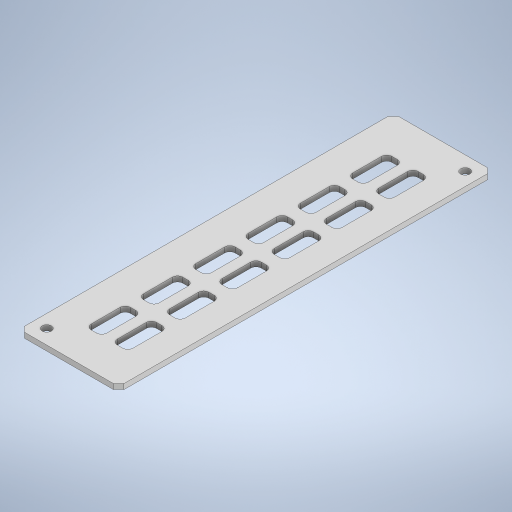
# Autodesk Inventor part: battery case Lid
Saved by Autodesk Inventor 2024 (Build 280153020, 153B)
## iProperties
Created: 2024-02-15
Part Number: battery case Lid
Material: Generic
Document SubType Name: Modeling
Designer: scottst
Density: 1 g/cm^3
Appearance: Default
Author: scottst
Autodesk Inventor part; units mm, degrees
ref_plane "YZ Plane" through (0, 0, 0) normal (1, 0, 0) x (0, 1, 0)
ref_plane "XZ Plane" through (0, 0, 0) normal (0, 1, 0) x (-1, 0, 0)
ref_plane "XY Plane" through (0, 0, 0) normal (0, 0, 1) x (1, 0, 0)
sketch "Sketch1" plane through (0, 0, 0) normal (0, 1, 0) x (-1, 0, 0)
  line L0 (-19, 71.5) -> (19, 71.5)
  line L1 (19, 71.5) -> (19, -71.5)
  line L2 (19, -71.5) -> (-19, -71.5)
  line L3 (-19, -71.5) -> (-19, 71.5)
  line L4 (-19, 71.5) -> (19, -71.5) construction
  line L5 (19, 71.5) -> (-19, -71.5) construction
  point P0 (0, 0)
  dimension "d0" = 38
  dimension "d1" = 143
  constraints: 12 end point, 2 midpoint, 2 parallel, 1 horizontal, 1 perpendicular
  measures "d0" distance of L1.end L2.end
  measures "d1" distance of L0.end L1.end
extrude "Extrusion1" add sketch "Sketch1" along normal blind 2
sketch "Sketch2" plane through (0, 2, 0) normal (0, 1, 0) x (1, 0, 0)
  line L0 (-19, -71.5) -> (-19, -66) construction
  line L1 (-19, -66) -> (-14, -66) construction
  line L2 (-19, -66) -> (-14, -66) construction
  line L3 (19, 71.5) -> (-19, 71.5) construction
  line L4 (19, 71.5) -> (19, 66) construction
  line L5 (19, 66) -> (14, 66) construction
  line L6 (19, 66) -> (24, 66) construction
  circle A0 centre (14, 66) radius 1.75
  circle A1 centre (-14, -66) radius 1.75
  point P0 (0, 0)
  dimension "d4" = 5.5
  dimension "d7" = 5
  dimension "d8" = 0
  dimension "d9" = 5.5
  dimension "d12" = 180
  dimension "d13" = 3.5
  dimension "d14" = 3.5
  constraints: 12 end point, 3 horizontal, 2 centre point, 2 coincident, 2 collinear
  measures "d4" distance of L0.start L0.end
  measures "d7" distance of L0.end L1.end
  measures "d8" distance between parallel lines of L1 L2
  measures "d9" distance of L3.start L4.end
  measures "d12" angle of L5 L6
  measures "d13" diameter of A0
  measures "d14" diameter of A1
extrude "Extrusion2" cut sketch "Sketch2" against normal blind 14.75
sketch "Sketch3" plane through (0, 0, 0) normal (0, -1, 0) x (1, 0, 0)
  line L0 (-14.75, 51.7235) -> (14.75, 51.7235)
  line L1 (14.75, 51.7235) -> (14.75, -51.7235)
  line L2 (14.75, -51.7235) -> (-14.75, -51.7235)
  line L3 (-14.75, -51.7235) -> (-14.75, 51.7235)
  line L4 (-14.75, 51.7235) -> (14.75, -51.7235) construction
  line L5 (14.75, 51.7235) -> (-14.75, -51.7235) construction
  line L6 (12.75, -49.7235) -> (12.75, 49.7235)
  line L7 (12.75, 49.7235) -> (-12.75, 49.7235)
  line L8 (-12.75, 49.7235) -> (-12.75, -49.7235)
  line L9 (-12.75, -49.7235) -> (12.75, -49.7235)
  line L10 (-14.75, 49.7235) -> (14.75, 49.7235)
  line L11 (-14.75, -49.7235) -> (14.75, -49.7235)
  line L12 (-14.75, 0) -> (-14.75, -25)
  line L13 (-14.75, -25) -> (14.75, -25)
  line L14 (-14.75, 0) -> (-14.75, 25)
  line L15 (-14.75, 25) -> (14.75, 25)
  point P0 (0, 0)
  point P1 (-12.75, -25)
  point P2 (12.75, -25)
  point P3 (12.75, 25)
  point P4 (-12.75, 25)
  dimension "d17" = 29.5
  dimension "d18" = 2
  dimension "d19" = 25
  dimension "d20" = 25
  constraints: 32 end point, 10 point on line, 4 parallel, 4 perpendicular, 3 midpoint, 1 horizontal, 3 other
  measures "d17" distance of L1.end L2.end
  measures "d18" distance between parallel lines of L1 L6
  measures "d19" distance of L12.start L12.end
  measures "d20" distance of L12.start L14.end
extrude "Extrusion3" add sketch "Sketch3" along normal blind 2 contours L10 L8 L15 L3 | L1 L15 L6 L10 | L1 L11 L6 L13 | L13 L8 L11 L3
sketch "Sketch4" plane through (0, 0, 0) normal (0, -1, 0) x (1, 0, 0)
  line L0 (-19, 71.5) -> (19, 71.5) construction
  line L1 (0, 71.5) -> (0, -71.5) construction
  line L2 (19, -71.5) -> (-19, -71.5) construction
  line L3 (3, 16) -> (3, 5) construction
  line L4 (-3, 71.5) -> (-3, -71.5) construction
  line L5 (-9, 71.5) -> (-9, -71.5) construction
  line L6 (9, 16) -> (9, -71.5) construction
  line L7 (19, 71.5) -> (19, -71.5) construction
  line L8 (19, 0) -> (-19, 0) construction
  line L9 (19, 3) -> (5, 3) construction
  line L10 (3, 3) -> (7, 3)
  line L11 (9, 5) -> (9, 18)
  line L12 (7, 18) -> (5, 18)
  line L13 (3, 18) -> (3, 3)
  arc A0 (5, 18) -> (3, 16) centre (5, 16) ccw
  arc A1 (9, 16) -> (7, 18) centre (7, 16) ccw
  arc A2 (7, 3) -> (9, 5) centre (7, 5) ccw
  arc A3 (3, 5) -> (5, 3) centre (5, 5) ccw
  point P0 (0, 0)
  point P1 (9, 3)
  dimension "d23" = 3
  dimension "d24" = 3
  dimension "d25" = 6
  dimension "d26" = 6
  dimension "d27" = 3
  dimension "d28" = 15
  dimension "d29" = 2
  constraints: 22 end point, 8 point on circle, 8 tangent, 7 parallel, 7 point on line, 4 centre point, 3 equal radius, 3 midpoint, 2 horizontal, 1 perpendicular
  measures "d23" distance between parallel lines of L1 L3
  measures "d24" distance between parallel lines of L1 L4
  measures "d25" distance between parallel lines of L4 L5
  measures "d26" distance between parallel lines of L3 L6
  measures "d27" distance between parallel lines of L8 L9
  measures "d28" distance of L11.end point (9, 3)
  measures "d29" radius of A0
extrude "Extrusion4" cut sketch "Sketch4" against normal blind 2 contours A3 L13 A0 L12 A1 L11 A2 L10
pattern_linear "Rectangular Pattern1" count 4 spacing 20 along (0, 0, -1) count 2 spacing 10 along (-1, 0, 0) of "Extrusion4"
pattern_linear "Rectangular Pattern2" count 3 spacing 20 along (0, 0, 1) count 2 spacing 10 along (-1, 0, 0) of "Extrusion4"
chamfer "Chamfer1" distance 2 angle 45 4 edges at (19, 1, -71.5) (-19, 1, -71.5) (-19, 1, 71.5) (19, 1, 71.5)
body "Solid1"
